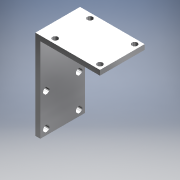
# Autodesk Inventor part: Pneumatic  Bottom Angled Plate
Saved by Autodesk Inventor 2019.4 (Build 234330000, 330)
## iProperties
Created: 2020-01-26
Part Number: Pneumatic  Bottom Angled Plate
Material: Aluminum 6061
Document SubType Name: Modeling
Designer: Mark
Mass: 25.5456 g
Surface Area: 50.9294 cm^2
Volume: 9.46134 cm^3
Density: 2.7 g/cm^3
Appearance: Aluminum - Flat
Author: Mark
Autodesk Inventor part; units mm, degrees
ref_plane "YZ Plane" through (0, 0, 0) normal (1, 0, 0) x (0, 1, 0)
ref_plane "XZ Plane" through (0, 0, 0) normal (0, 1, 0) x (-1, 0, 0)
ref_plane "XY Plane" through (0, 0, 0) normal (0, 0, 1) x (1, 0, 0)
sketch "Sketch1" plane through (0, 0, 0) normal (1, 0, 0) x (0, 1, 0)
  line L0 (-22.5, 22.5) -> (22.5, 22.5)
  line L1 (22.5, 22.5) -> (22.5, -22.5)
  line L2 (22.5, -22.5) -> (-22.5, -22.5)
  line L3 (-22.5, -22.5) -> (-22.5, 22.5)
  line L4 (-22.5, 22.5) -> (22.5, -22.5) construction
  line L5 (22.5, 22.5) -> (-22.5, -22.5) construction
  line L6 (-16.5, 16.5) -> (16.5, 16.5) construction
  line L7 (16.5, 16.5) -> (16.5, -16.5) construction
  line L8 (16.5, -16.5) -> (-16.5, -16.5) construction
  line L9 (-16.5, -16.5) -> (-16.5, 16.5) construction
  line L10 (-16.5, 16.5) -> (16.5, -16.5) construction
  line L11 (16.5, 16.5) -> (-16.5, -16.5) construction
  circle A0 centre (16.5, 16.5) radius 3.25
  circle A1 centre (16.5, -16.5) radius 3.25
  circle A2 centre (-16.5, -16.5) radius 3.25
  circle A3 centre (-16.5, 16.5) radius 3.25
  line L12 (22.5, 22.5) -> (67.5, 22.5)
  line L13 (67.5, 22.5) -> (67.5, -22.5)
  line L14 (67.5, -22.5) -> (22.5, -22.5)
  line L15 (22.5, -22.5) -> (22.5, 22.5)
  point P0 (0, 0)
  dimension "d0" = 45
  dimension "d1" = 45
  dimension "d2" = 33
  dimension "d3" = 33
  dimension "d4" = 6.5
  dimension "d5" = 6.5
  dimension "d6" = 6.5
  dimension "d7" = 6.5
  dimension "d30" = 45
  dimension "d31" = 45
  constraints: 32 end point, 6 parallel, 4 centre point, 4 coincident, 4 midpoint, 3 horizontal, 3 perpendicular
  measures "d0" distance of L1.end L2.end
  measures "d1" distance of L0.end L1.end
  measures "d2" distance of L7.end L8.end
  measures "d3" distance of L6.end L7.end
  measures "d4" diameter of A0
  measures "d5" diameter of A1
  measures "d6" diameter of A2
  measures "d7" diameter of A3
  measures "d30" distance of L13.end L14.end
  measures "d31" distance of L12.end L13.end
extrude "Extrusion1" add sketch "Sketch1" along normal blind 5
sketch "Sketch2" plane through (5, 0, 0) normal (1, 0, 0) x (0, 0, -1)
  line L0 (-22.5, 67.5) -> (-22.5, -22.5) projected
  line L1 (-22.5, 62.5) -> (22.5, 62.5)
  line L2 (22.5, 62.5) -> (22.5, 67.5)
  line L3 (22.5, 67.5) -> (-22.5, 67.5)
  line L4 (-22.5, 67.5) -> (-22.5, 62.5)
  line L5 (22.5, 67.5) -> (-22.5, 67.5) projected
  point P0 (0, 0)
  dimension "d10" = 45
  dimension "d11" = 5
  constraints: 8 end point, 2 collinear, 2 parallel, 1 horizontal, 1 perpendicular
  measures "d10" distance of L3.end L2.end
  measures "d11" distance of L2.end L1.end
extrude "Extrusion2" add sketch "Sketch2" along normal blind 60 and the other way blind 5
sketch "Sketch3" plane through (5, 62.5, -22.5) normal (0, -1, 0) x (1, 0, 0)
  circle A0 centre (10, 40) radius 2.75
  circle A1 centre (55, 40) radius 2.75
  circle A2 centre (10, 5) radius 2.75
  circle A3 centre (55, 5) radius 2.75
  line L0 (0, 0) -> (60, 0) projected
  line L1 (60, 45) -> (60, 0) projected
  line L2 (60, 45) -> (0, 45) projected
  line L3 (-5, 0) -> (-5, 45) projected
  point P0 (-5, 22.5)
  dimension "d16" = 5.5
  dimension "d17" = 5.5
  dimension "d18" = 5.5
  dimension "d19" = 5.5
  dimension "d20" = 5
  dimension "d21" = 5
  dimension "d22" = 5
  dimension "d23" = 5
  dimension "d24" = 5
  dimension "d25" = 15
  dimension "d26" = 15
  dimension "d27" = 5
  constraints: 4 centre point
  measures "d16" diameter of A0
  measures "d17" diameter of A1
  measures "d18" diameter of A2
  measures "d19" diameter of A3
  measures "d20" distance from line of L0 A3.centre
  measures "d21" distance from line of L1 A3.centre
  measures "d22" distance from line of L1 A1.centre
  measures "d23" distance from line of L2 A1.centre
  measures "d24" distance from line of L2 A0.centre
  measures "d25" distance from line of L3 A0.centre
  measures "d26" distance from line of L3 A2.centre
  measures "d27" distance from line of L0 A2.centre
extrude "Extrusion3" cut sketch "Sketch3" against normal up to next
body "Solid1"
